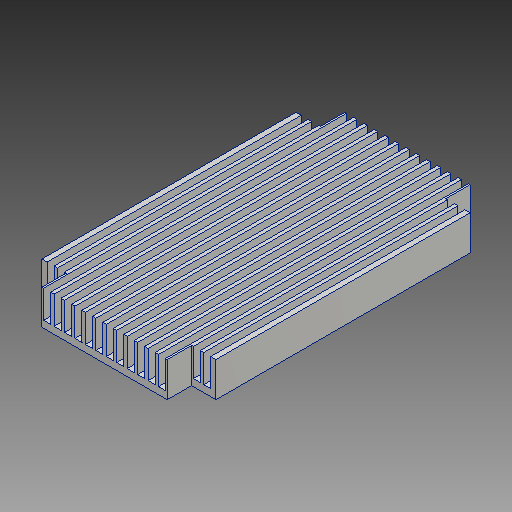
# Autodesk Inventor part: Jetson Kühlkörper Original
Saved by Autodesk Inventor 2019.1 (Build 231200000, 200)
## iProperties
Part Number: Jetson Kühlkörper Original
Material: Aluminium 6061
Document SubType Name: Modeling
Designer: rYan
Mass: 54.4428 g
Surface Area: 319.12 cm^2
Volume: 20.164 cm^3
Density: 2.7 g/cm^3
Appearance: Aluminium - flach
Author: rYan
Autodesk Inventor part; units mm, degrees
ref_plane "YZ Plane" through (0, 0, 0) normal (1, 0, 0) x (0, 1, 0)
ref_plane "XZ Plane" through (0, 0, 0) normal (0, 1, 0) x (-1, 0, 0)
ref_plane "XY Plane" through (0, 0, 0) normal (0, 0, 1) x (1, 0, 0)
sketch "Skizze1" plane through (0, 0, 0) normal (0, 0, 1) x (1, 0, 0)
  line L0 (-18, 43.5) -> (18, 43.5)
  line L1 (25, 36.5) -> (25, -36.5)
  line L2 (18, -43.5) -> (-18, -43.5)
  line L3 (-25, -36.5) -> (-25, 36.5)
  line L4 (-18, 43.5) -> (-18, 36.5)
  line L5 (-18, 36.5) -> (-25, 36.5)
  line L6 (18, 43.5) -> (18, 36.5)
  line L7 (18, 36.5) -> (25, 36.5)
  line L8 (-18, -43.5) -> (-18, -36.5)
  line L9 (-18, -36.5) -> (-25, -36.5)
  line L10 (18, -43.5) -> (18, -36.5)
  line L11 (18, -36.5) -> (25, -36.5)
  line L12 (0, 60.9) -> (0, -60.9) projected
  line L13 (-35, 0) -> (35, 0) projected
  point P0 (0, 0)
  dimension "d6" = 87
  dimension "d7" = 50
  dimension "d8" = 7
  dimension "d9" = 7
  constraints: 24 end point, 4 point on line, 2 parallel, 1 horizontal, 1 perpendicular, 1 vertical, 7 other
  measures "d6" distance between parallel lines of L2 L0
  measures "d7" distance between parallel lines of L1 L3
  measures "d8" distance of L4.end L3.end
  measures "d9" distance of L0.start L4.end
extrude "Extrusion1" add sketch "Skizze1" along normal blind 10
sketch "Skizze2" plane through (0, 0, 10) normal (0, 0, 1) x (1, 0, 0)
  line L0 (-18, -43.5) -> (18, -43.5) projected
  line L1 (18, -43.5) -> (18, -36.5) projected
  line L2 (18, -36.5) -> (25, -36.5) projected
  line L3 (25, -36.5) -> (25, 36.5) projected
  line L4 (25, 36.5) -> (18, 36.5) projected
  line L5 (18, 36.5) -> (18, 43.5) projected
  line L6 (18, 43.5) -> (-18, 43.5) projected
  line L7 (-18, 43.5) -> (-18, 36.5) projected
  line L8 (-18, 36.5) -> (-25, 36.5) projected
  line L9 (-25, 36.5) -> (-25, -36.5) projected
  line L10 (-25, -36.5) -> (-18, -36.5) projected
  line L11 (-18, -36.5) -> (-18, -43.5) projected
  line L12 (-23.5, 43.5) -> (-21.5, 43.5)
  line L13 (-21.5, 43.5) -> (-21.5, -43.5)
  line L14 (-21.5, -43.5) -> (-23.5, -43.5)
  line L15 (-23.5, -43.5) -> (-23.5, 43.5)
  line L16 (-18, -43.5) -> (18, -43.5) projected
  point P0 (0, 0)
  dimension "d12" = 1.5
  dimension "d13" = 2
  constraints: 8 end point, 2 parallel, 1 collinear, 1 horizontal, 1 perpendicular, 1 point on line
  measures "d12" distance between parallel lines of L9 L15
  measures "d13" distance of L12.start L12.end
extrude "Extrusion2" cut sketch "Skizze2" against normal blind 8 contours L13 L14 L15 L10 | L10 L15 L8 L13 | L8 L15 L12 L13
pattern_linear "Rechteckige Anordnung1" count 16 spacing 3 along (1, 0, 0) of "Extrusion2"
